omniwheel_rim (Autodesk Fusion 360 design; units mm, degrees)
part number: 2026-09-20-21-30-31-759
Autodesk Fusion 360 part; units mm, degrees
sketch "Sketch3" plane through (0, 0, 0) normal (0, 0, 1) x (1, 0, 0)
  circle A0 centre (-50, 25) radius 27.5
  line L0 (-40.5, 45) -> (-40.5, 60)
  line L1 (-59.5, 60) -> (-59.5, 45)
  line L2 (-50, 25) -> (-50, 55)
  circle A1 centre (-50, 25) radius 16.25
  spline S0 degree 2 poles (-59.5, 45) (-50.3564, 40) (-40.5, 45) knots 0 0 0 2.042764 2.042764 2.042764 weights 1 3 1
  dimension "d9" = 55
  dimension "d10" = 32.5
  constraint vertical L0
  constraint coincident A0.centre L2.start
  constraint vertical L2
  constraint concentric A0 A1
  measures "d9" diameter of A0
  measures "d10" diameter of A1
extrude "Extrude3" add sketch "Sketch3" along normal blind 5
sketch "Sketch4" plane through (0, 0, 5) normal (0, 0, 1) x (-1, 0, 0)
  circle A0 centre (50, -25) radius 27.5
  line L0 (50, -25) -> (50, -61)
  line L1 (59.5, -45) -> (59.5, -62)
  line L2 (40.5, -62) -> (40.5, -45)
  circle A1 centre (50, -25) radius 16.25
  spline S0 degree 2 poles (59.5, -45) (50, -40) (40.5, -45) knots 0 0 0 2.04267 2.04267 2.04267 weights 1 3 1
  line L3 (82.2534, -45.4687) -> (66.0855, -40.2154)
  spline S1 degree 2 poles (71.9568, -22.1453) (64.2658, -29.6353) (66.0855, -40.2154) knots 0 0 0 2.04267 2.04267 2.04267 weights 1 3 1
  line L4 (71.9568, -22.1453) -> (88.1248, -27.3986)
  line L5 (50, -25) -> (84.238, -36.1246)
  line L6 (79.4337, -0.6503) -> (69.4414, -14.4036)
  spline S2 degree 2 poles (54.07, -3.2357) (58.8168, -12.8647) (69.4414, -14.4036) knots 0 0 0 2.04267 2.04267 2.04267 weights 1 3 1
  line L7 (54.07, -3.2357) -> (64.0624, 10.5176)
  line L8 (50, -25) -> (71.1603, 4.1246)
  line L9 (35.9376, 10.5176) -> (45.93, -3.2357)
  spline S3 degree 2 poles (30.5586, -14.4036) (41.1832, -12.8647) (45.93, -3.2357) knots 0 0 0 2.04267 2.04267 2.04267 weights 1 3 1
  line L10 (30.5586, -14.4036) -> (20.5663, -0.6503)
  line L11 (50, -25) -> (28.8397, 4.1246)
  line L12 (11.8752, -27.3986) -> (28.0432, -22.1453)
  spline S4 degree 2 poles (33.9145, -40.2154) (35.7342, -29.6353) (28.0432, -22.1453) knots 0 0 0 2.04267 2.04267 2.04267 weights 1 3 1
  line L13 (33.9145, -40.2154) -> (17.7466, -45.4687)
  line L14 (50, -25) -> (15.762, -36.1246)
  dimension "d14" = 32.5
  dimension "d21" = 360
  constraint coincident A0.centre L0.start
  constraint vertical L0
  constraint vertical L1
  measures "d14" diameter of A1
extrude "Extrude4" cut sketch "Sketch4" against normal blind 30 contours A0 S1 L4 L5 | A0 L3 S1 L5 | A0 L6 S2 L8 | A0 S2 L7 L8 | A0 L0 L1 S0 | A0 L0 L2 S0 | A0 L12 S4 L14 | A0 S4 L13 L14 | A0 L9 S3 L11 | A0 S3 L10 L11
sketch "Sketch5" plane through (0, 0, 5) normal (0, 0, 1) x (-1, 0, 0)
  line L0 (71.9568, -22.1453) -> (77.4796, -23.9398)
  arc A0 (77.4796, -23.9398) -> (72.8546, -9.7057) centre (50, -25) ccw
  line L1 (72.8546, -9.7057) -> (69.4414, -14.4036)
  spline S0 degree 2 poles (69.4414, -14.4036) (58.8168, -12.8647) (54.07, -3.2357) knots -2.04267 -2.04267 -2.04267 0 0 0 weights 1 3 1
  line L2 (54.07, -3.2357) -> (57.4833, 1.4622)
  arc A1 (57.4833, 1.4622) -> (42.5167, 1.4622) centre (50, -25) ccw
  line L3 (42.5167, 1.4622) -> (45.93, -3.2357)
  spline S1 degree 2 poles (45.93, -3.2357) (41.1832, -12.8647) (30.5586, -14.4036) knots -2.04267 -2.04267 -2.04267 0 0 0 weights 1 3 1
  line L4 (30.5586, -14.4036) -> (27.1454, -9.7057)
  arc A2 (27.1454, -9.7057) -> (22.5204, -23.9398) centre (50, -25) ccw
  line L5 (22.5204, -23.9398) -> (28.0432, -22.1453)
  spline S2 degree 2 poles (28.0432, -22.1453) (35.7342, -29.6353) (33.9145, -40.2154) knots -2.04267 -2.04267 -2.04267 0 0 0 weights 1 3 1
  line L6 (33.9145, -40.2154) -> (28.3918, -42.0098)
  arc A3 (28.3918, -42.0098) -> (40.5, -50.807) centre (50, -25) ccw
  line L7 (40.5, -50.807) -> (40.5, -45)
  spline S3 degree 2 poles (40.5, -45) (50, -40) (59.5, -45) knots -2.04267 -2.04267 -2.04267 0 0 0 weights 1 3 1
  line L8 (59.5, -45) -> (59.5, -50.807)
  arc A4 (59.5, -50.807) -> (71.6082, -42.0098) centre (50, -25) ccw
  line L9 (71.6082, -42.0098) -> (66.0855, -40.2154)
  spline S4 degree 2 poles (66.0855, -40.2154) (64.2658, -29.6353) (71.9568, -22.1453) knots -2.04267 -2.04267 -2.04267 0 0 0 weights 1 3 1
  circle A5 centre (50, -25) radius 10
  circle A6 centre (50, -35) radius 1.5
  circle A7 centre (58.6603, -30) radius 1.5
  circle A8 centre (58.6603, -20) radius 1.5
  circle A9 centre (50, -15) radius 1.5
  circle A10 centre (41.3397, -20) radius 1.5
  circle A11 centre (41.3397, -30) radius 1.5
  circle A12 centre (50, -25) radius 6
  line L10 (50, -25) -> (33.8359, -47.248)
  circle A13 centre (35.5881, -44.8363) radius 1.5
  circle A14 centre (64.4119, -44.8363) radius 1.5
  circle A15 centre (73.319, -17.4232) radius 1.5
  circle A16 centre (50, -0.481) radius 1.5
  circle A17 centre (26.681, -17.4232) radius 1.5
  dimension "d24" = 20
  dimension "d25" = 3
  dimension "d27" = 360
  dimension "d28" = 3
  dimension "d30" = 360
  constraint concentric A0 A5
  constraint coincident A5 A6.centre
  constraint concentric A0 A12
  constraint coincident A0.centre A1.centre
  constraint midpoint A3 L10.end
  constraint coincident L10 A13.centre
  measures "d24" diameter of A5
  measures "d25" diameter of A6
  measures "d28" diameter of A13
extrude "Extrude5" cut sketch "Sketch5" against normal blind 5 contours A5 A8 | A5 A8 | A5 A7 | A5 A7 | A5 A9 | A5 A9 | A5 A6 | A5 A6 | A5 A10 | A5 A10 | A5 A11 | A5 A11 | A12 | L10 A13 | L10 A13 | A14 | A15 | A16 | A17
sketch "Sketch6" plane through (0, 0, 5) normal (0, 0, 1) x (-1, 0, 0)
  line L0 (71.9568, -22.1453) -> (77.4796, -23.9398)
  arc A0 (77.4796, -23.9398) -> (72.8546, -9.7057) centre (50, -25) ccw
  line L1 (72.8546, -9.7057) -> (69.4414, -14.4036)
  spline S0 degree 2 poles (69.4414, -14.4036) (58.8168, -12.8647) (54.07, -3.2357) knots -2.04267 -2.04267 -2.04267 0 0 0 weights 1 3 1
  line L2 (54.07, -3.2357) -> (57.4833, 1.4622)
  arc A1 (57.4833, 1.4622) -> (42.5167, 1.4622) centre (50, -25) ccw
  line L3 (42.5167, 1.4622) -> (45.93, -3.2357)
  spline S1 degree 2 poles (45.93, -3.2357) (41.1832, -12.8647) (30.5586, -14.4036) knots -2.04267 -2.04267 -2.04267 0 0 0 weights 1 3 1
  line L4 (30.5586, -14.4036) -> (27.1454, -9.7057)
  arc A2 (27.1454, -9.7057) -> (22.5204, -23.9398) centre (50, -25) ccw
  line L5 (22.5204, -23.9398) -> (28.0432, -22.1453)
  spline S2 degree 2 poles (28.0432, -22.1453) (35.7342, -29.6353) (33.9145, -40.2154) knots -2.04267 -2.04267 -2.04267 0 0 0 weights 1 3 1
  line L6 (33.9145, -40.2154) -> (28.3918, -42.0098)
  arc A3 (28.3918, -42.0098) -> (40.5, -50.807) centre (50, -25) ccw
  line L7 (40.5, -50.807) -> (40.5, -45)
  spline S3 degree 2 poles (40.5, -45) (50, -40) (59.5, -45) knots -2.04267 -2.04267 -2.04267 0 0 0 weights 1 3 1
  line L8 (59.5, -45) -> (59.5, -50.807)
  arc A4 (59.5, -50.807) -> (71.6082, -42.0098) centre (50, -25) ccw
  line L9 (71.6082, -42.0098) -> (66.0855, -40.2154)
  spline S4 degree 2 poles (66.0855, -40.2154) (64.2658, -29.6353) (71.9568, -22.1453) knots -2.04267 -2.04267 -2.04267 0 0 0 weights 1 3 1
  circle A5 centre (50, -0.481) radius 1.5
  circle A6 centre (35.5881, -44.8363) radius 1.5
  circle A7 centre (58.6603, -30) radius 1.5
  circle A8 centre (50, -25) radius 6
  circle A9 centre (58.6603, -20) radius 1.5
  circle A10 centre (64.4119, -44.8363) radius 1.5
  circle A11 centre (26.681, -17.4232) radius 1.5
  circle A12 centre (41.3397, -20) radius 1.5
  circle A13 centre (50, -35) radius 1.5
  circle A14 centre (41.3397, -30) radius 1.5
  circle A15 centre (50, -15) radius 1.5
  circle A16 centre (73.319, -17.4232) radius 1.5
  circle A17 centre (50, -25) radius 14
  dimension "d33" = 28
  constraint concentric A0 A17
  measures "d33" diameter of A17
extrude "Extrude6" cut sketch "Sketch6" against normal blind 1.5 contours A17
sketch "Sketch7" plane through (0, 0, 5) normal (0, 0, 1) x (-1, 0, 0)
  circle A0 centre (73.319, -17.4232) radius 1.5
  circle A1 centre (26.681, -17.4232) radius 1.5
  circle A2 centre (64.4119, -44.8363) radius 1.5
  circle A3 centre (35.5881, -44.8363) radius 1.5
  circle A4 centre (50, -0.481) radius 1.5
  line L0 (71.9568, -22.1453) -> (77.4796, -23.9398)
  arc A5 (77.4796, -23.9398) -> (72.8546, -9.7057) centre (50, -25) ccw
  line L1 (72.8546, -9.7057) -> (69.4414, -14.4036)
  spline S0 degree 2 poles (69.4414, -14.4036) (58.8168, -12.8647) (54.07, -3.2357) knots -2.04267 -2.04267 -2.04267 0 0 0 weights 1 3 1
  line L2 (54.07, -3.2357) -> (57.4833, 1.4622)
  arc A6 (57.4833, 1.4622) -> (42.5167, 1.4622) centre (50, -25) ccw
  line L3 (42.5167, 1.4622) -> (45.93, -3.2357)
  spline S1 degree 2 poles (45.93, -3.2357) (41.1832, -12.8647) (30.5586, -14.4036) knots -2.04267 -2.04267 -2.04267 0 0 0 weights 1 3 1
  line L4 (30.5586, -14.4036) -> (27.1454, -9.7057)
  arc A7 (27.1454, -9.7057) -> (22.5204, -23.9398) centre (50, -25) ccw
  line L5 (22.5204, -23.9398) -> (28.0432, -22.1453)
  spline S2 degree 2 poles (28.0432, -22.1453) (35.7342, -29.6353) (33.9145, -40.2154) knots -2.04267 -2.04267 -2.04267 0 0 0 weights 1 3 1
  line L6 (33.9145, -40.2154) -> (28.3918, -42.0098)
  arc A8 (28.3918, -42.0098) -> (40.5, -50.807) centre (50, -25) ccw
  line L7 (40.5, -50.807) -> (40.5, -45)
  spline S3 degree 2 poles (40.5, -45) (50, -40) (59.5, -45) knots -2.04267 -2.04267 -2.04267 0 0 0 weights 1 3 1
  line L8 (59.5, -45) -> (59.5, -50.807)
  arc A9 (59.5, -50.807) -> (71.6082, -42.0098) centre (50, -25) ccw
  line L9 (71.6082, -42.0098) -> (66.0855, -40.2154)
  spline S4 degree 2 poles (66.0855, -40.2154) (64.2658, -29.6353) (71.9568, -22.1453) knots -2.04267 -2.04267 -2.04267 0 0 0 weights 1 3 1
  circle A10 centre (50, -25) radius 14
  line L10 (61, -48) -> (39, -48)
  line L11 (50, -25) -> (50, -48)
  line L12 (61, -49) -> (39, -49)
  line L13 (39, -49) -> (39, -48)
  line L14 (61, -49) -> (61, -48)
  line L15 (75.2735, -21.6458) -> (68.4751, -42.569)
  line L16 (76.2245, -21.9548) -> (75.2735, -21.6458)
  line L17 (76.2245, -21.9548) -> (69.4262, -42.878)
  line L18 (69.4262, -42.878) -> (68.4751, -42.569)
  line L19 (54.6199, 0.073) -> (72.4182, -12.8582)
  line L20 (55.2077, 0.882) -> (54.6199, 0.073)
  line L21 (55.2077, 0.882) -> (73.006, -12.0492)
  line L22 (73.006, -12.0492) -> (72.4182, -12.8582)
  line L23 (27.5818, -12.8582) -> (45.3801, 0.073)
  line L24 (26.994, -12.0492) -> (27.5818, -12.8582)
  line L25 (26.994, -12.0492) -> (44.7923, 0.882)
  line L26 (44.7923, 0.882) -> (45.3801, 0.073)
  line L27 (31.5249, -42.569) -> (24.7265, -21.6458)
  line L28 (30.5738, -42.878) -> (31.5249, -42.569)
  line L29 (30.5738, -42.878) -> (23.7755, -21.9548)
  line L30 (23.7755, -21.9548) -> (24.7265, -21.6458)
  dimension "d37" = 360
  constraint horizontal L10
  constraint coincident A5.centre A6.centre
  constraint midpoint L10 L11.end
  constraint perpendicular L7 L12
  constraint perpendicular L10 L13
  constraint perpendicular L10 L14
extrude "Extrude7" cut sketch "Sketch7" against normal blind 1.5 contours L0 L15 L16 L17 | L9 L15 L17 L18 | L1 L19 L21 L22 | L2 L19 L20 L21 | L8 L10 L12 L14 | L7 L10 L12 L13 | L3 L23 L25 L26 | L4 L23 L24 L25 | L6 L27 L28 L29 | L5 L27 L29 L30
sketch "Sketch1" plane through (0, 0, 0) normal (0, 0, 1) x (1, 0, 0)
  circle A0 centre (-75, 50) radius 40
extrude "Extrude1" [suppressed]
sketch "Sketch2" plane through (0, 0, 40) normal (0, 0, 1) x (-1, 0, 0)
  circle A0 centre (75, -50) radius 40
  circle A1 centre (75, -50) radius 30
  line L0 (75, -50) -> (56.4216, -73.5551)
  line L1 (75, -50) -> (93.5784, -73.5551)
  line L2 (75, -50) -> (93.5784, -26.4449)
  line L3 (56.4216, -26.0914) -> (75, -50)
  constraint concentric A0 A1
  constraint coincident A0.centre A1.centre
  constraint coincident A1 L0.end
  constraint coincident A1 L1.end
  constraint coincident A1 L2.end
  constraint parallel L0 L2
extrude "Extrude2" [suppressed]
fillet "Fillet1" [suppressed]
fillet "Fillet2" [suppressed]
equation "d15 = 0.75"
equation "d16 = d15"
equation "d17 = d15"
equation "d18 = d15"
equation "d19 = d15"
